Autodesk Inventor part; units mm, degrees
(part 2 of 2)
  spline S317 degree 2 poles (4.7592, -20.8202) (4.7075, -20.8826) (4.5777, -20.9876) knots 0 0 0 1 1 1
  line L179 (4.5777, -20.9876) -> (6.0592, -20.5763)
  spline S318 degree 2 poles (6.0592, -20.5763) (6.2625, -20.5199) (6.4389, -20.3989) (6.5028, -20.1862) (6.4937, -19.9698) knots 0 0 0 1 2 3 3 3
  line L180 (6.4937, -19.9698) -> (6.4825, -19.778)
  line L181 (6.4825, -19.778) -> (6.6607, -19.7285)
  spline S319 degree 2 poles (8.7637, -20.3753) (8.3867, -20.5516) (7.5473, -20.4146) (6.8295, -19.8283) (6.6188, -19.378) knots 0 0 0 1 2 3 3 3
  spline S320 degree 2 poles (6.6188, -19.378) (6.4106, -18.933) (6.4141, -18.006) (6.8248, -17.281) (7.2018, -17.1047) knots 0 0 0 1 2 3 3 3
  spline S321 degree 2 poles (7.2018, -17.1047) (7.3484, -17.0361) (7.7003, -16.9768) (8.0756, -17.015) (8.2787, -17.1082) knots 0 0 0 1 2 3 3 3
  spline S322 degree 2 poles (8.2787, -17.1082) (8.5842, -17.1951) (9.1378, -17.7306) (9.3178, -18.1154) knots 0 0 0 1 2 2 2
  spline S323 degree 2 poles (9.3178, -18.1154) (9.4281, -18.351) (9.5371, -18.8297) (9.5213, -19.287) (9.3843, -19.7308) (9.2645, -19.9112) knots 0 0 0 1 2 3 4 4 4
  spline S324 degree 2 poles (9.2645, -19.9112) (9.0516, -20.2406) (8.7637, -20.3753) knots 0 0 0 1 1 1
  line L182 (7.3086, -18.7108) -> (7.5755, -19.2815)
  spline S325 degree 2 poles (7.5755, -19.2815) (7.867, -19.9045) (8.3959, -20.3463) (8.6603, -20.2226) knots 0 0 0 1 2 2 2
  spline S326 degree 2 poles (8.6603, -20.2226) (9.1865, -19.9764) (8.6759, -18.8848) knots 0 0 0 1 1 1
  line L183 (8.6759, -18.8848) -> (8.4003, -18.2958)
  spline S327 degree 2 poles (8.4003, -18.2958) (8.2827, -18.0444) (8.0517, -17.6324) (7.9802, -17.5478) knots 0 0 0 1 2 2 2
  spline S328 degree 2 poles (7.9802, -17.5478) (7.6465, -17.1072) (7.28, -17.2787) knots 0 0 0 1 1 1
  spline S329 degree 2 poles (7.28, -17.2787) (7.0967, -17.3644) (6.978, -17.704) (7.1028, -18.271) (7.3086, -18.7108) knots 0 0 0 1 2 3 3 3
  line L184 (11.9387, -16.7133) -> (12.5299, -18.012)
  line L185 (12.5299, -18.012) -> (10.3324, -19.5294)
  spline S330 degree 2 poles (10.3324, -19.5294) (10.1686, -19.2668) (10.2153, -18.8411) knots 0 0 0 1 1 1
  spline S331 degree 2 poles (10.2153, -18.8411) (10.2457, -18.5392) (10.5063, -17.8078) knots 0 0 0 1 1 1
  spline S332 degree 2 poles (10.5063, -17.8078) (10.6457, -17.4094) (10.6659, -17.3217) knots 0 0 0 1 1 1
  spline S333 degree 2 poles (10.6659, -17.3217) (10.6697, -17.312) (10.6809, -17.2621) (10.6898, -17.2139) knots 0 0 0 1 2 2 2
  spline S334 degree 2 poles (10.6898, -17.2139) (10.7351, -16.9438) (10.6498, -16.5355) (10.5135, -16.3381) knots 0 0 0 1 2 2 2
  spline S335 degree 2 poles (10.5135, -16.3381) (10.282, -16.0028) (9.7155, -15.8742) (9.4182, -16.0795) knots 0 0 0 1 2 2 2
  spline S336 degree 2 poles (9.4182, -16.0795) (9.1875, -16.2388) (8.932, -16.6927) (8.9316, -17.1601) (9.0613, -17.348) knots 0 0 0 1 2 3 3 3
  spline S337 degree 2 poles (9.0613, -17.348) (9.1845, -17.5263) (9.2392, -17.4886) knots 0 0 0 1 1 1
  spline S338 degree 2 poles (9.2392, -17.4886) (9.2416, -17.4869) (9.2242, -17.4567) knots 0 0 0 1 1 1
  spline S339 degree 2 poles (9.2242, -17.4567) (9.1985, -17.4042) (9.1838, -17.3371) knots 0 0 0 1 1 1
  spline S340 degree 2 poles (9.1838, -17.3371) (9.148, -17.1581) (9.2472, -16.9) (9.3851, -16.8047) knots 0 0 0 1 2 2 2
  spline S341 degree 2 poles (9.3851, -16.8047) (9.4993, -16.7259) (9.7514, -16.6993) (9.9737, -16.8127) (10.0476, -16.9198) knots 0 0 0 1 2 3 3 3
  spline S342 degree 2 poles (10.0476, -16.9198) (10.1347, -17.0458) (10.1482, -17.335) (10.013, -17.597) (9.8798, -17.6889) knots 0 0 0 1 2 3 3 3
  spline S343 degree 2 poles (9.8798, -17.6889) (9.6349, -17.8581) (9.0877, -17.7372) (8.9087, -17.4779) knots 0 0 0 1 2 2 2
  spline S344 degree 2 poles (8.9087, -17.4779) (8.802, -17.3233) (8.7156, -16.9439) (8.7696, -16.717) knots 0 0 0 1 2 2 2
  spline S345 degree 2 poles (8.7696, -16.717) (8.8426, -16.2276) (9.468, -15.7956) knots 0 0 0 1 1 1
  spline S346 degree 2 poles (9.468, -15.7956) (9.7249, -15.6183) (10.2567, -15.4372) (10.7436, -15.4557) (11.1422, -15.6616) (11.2719, -15.8495) knots 0 0 0 1 2 3 4 4 4
  spline S347 degree 2 poles (11.2719, -15.8495) (11.4657, -16.1301) (11.422, -16.494) knots 0 0 0 1 1 1
  spline S348 degree 2 poles (11.422, -16.494) (11.4098, -16.6289) (11.3538, -16.787) knots 0 0 0 1 1 1
  spline S349 degree 2 poles (11.3538, -16.787) (11.2506, -17.0444) (10.973, -17.4714) knots 0 0 0 1 1 1
  spline S350 degree 2 poles (10.973, -17.4714) (10.5939, -18.0669) (10.4994, -18.3675) knots 0 0 0 1 1 1
  spline S351 degree 2 poles (10.4994, -18.3675) (10.471, -18.4433) (10.3827, -18.585) knots 0 0 0 1 1 1
  line L186 (10.3827, -18.585) -> (11.6479, -17.7113)
  spline S352 degree 2 poles (11.6479, -17.7113) (11.8215, -17.5914) (11.9486, -17.4194) (11.9394, -17.1975) (11.8599, -16.9959) knots 0 0 0 1 2 3 3 3
  line L187 (11.8599, -16.9959) -> (11.7864, -16.8184)
  line L188 (11.7864, -16.8184) -> (11.9387, -16.7133)
  spline S353 degree 2 poles (14.1375, -16.6358) (13.839, -16.9259) (13.001, -17.0713) (12.1308, -16.7523) (11.7843, -16.3959) knots 0 0 0 1 2 3 3 3
  spline S354 degree 2 poles (11.7843, -16.3959) (11.4419, -16.0435) (11.1417, -15.1665) (11.2923, -14.347) (11.5908, -14.057) knots 0 0 0 1 2 3 3 3
  spline S355 degree 2 poles (11.5908, -14.057) (11.7068, -13.9442) (12.0199, -13.7728) (12.387, -13.6861) (12.6095, -13.7077) knots 0 0 0 1 2 3 3 3
  spline S356 degree 2 poles (12.6095, -13.7077) (12.9266, -13.6897) (13.625, -14.0144) (13.9211, -14.3191) knots 0 0 0 1 2 2 2
  spline S357 degree 2 poles (13.9211, -14.3191) (14.1024, -14.5056) (14.3622, -14.9222) (14.497, -15.3594) (14.5129, -15.8236) (14.4588, -16.0334) knots 0 0 0 1 2 3 4 4 4
  spline S358 degree 2 poles (14.4588, -16.0334) (14.3655, -16.4142) (14.1375, -16.6358) knots 0 0 0 1 1 1
  line L189 (12.2176, -15.5395) -> (12.6567, -15.9913)
  spline S359 degree 2 poles (12.6567, -15.9913) (13.1361, -16.4846) (13.7805, -16.7288) (13.9898, -16.5254) knots 0 0 0 1 2 2 2
  spline S360 degree 2 poles (13.9898, -16.5254) (14.4064, -16.1205) (13.5665, -15.2562) knots 0 0 0 1 1 1
  line L190 (13.5665, -15.2562) -> (13.1132, -14.7899)
  spline S361 degree 2 poles (13.1132, -14.7899) (12.9199, -14.5909) (12.5666, -14.2773) (12.4714, -14.2208) knots 0 0 0 1 2 2 2
  spline S362 degree 2 poles (12.4714, -14.2208) (12.0118, -13.9138) (11.7216, -14.1958) knots 0 0 0 1 1 1
  spline S363 degree 2 poles (11.7216, -14.1958) (11.5766, -14.3368) (11.5755, -14.6965) (11.8791, -15.1913) (12.2176, -15.5395) knots 0 0 0 1 2 3 3 3
  point P0 (0, 0)
  point P1 (-50, 12.5)
  point P2 (-50, -12.5)
  dimension "d18" = 47.5
  dimension "d19" = 95
  constraints: 6 end point, 4 point on circle, 2 centre point, 2 horizontal, 2 other
  measures "d18" distance of L2.start L2.end
  measures "d19" distance of L2.end L3.end
extrude "Extrusion3" add sketch "Skizze3" against normal blind 2 from surface at -3
extrude "Extrusion4" add sketch "Skizze4" along normal blind 2
ref_plane "Arbeitsebene1" through (0, 0, 3) normal (0, 0, 1) x (1, 0, 0)
sketch "Skizze5" plane through (0, 0, 3) normal (0, 0, 1) x (1, 0, 0)
  line L0 (-8.4237, 9.7925) -> (8.4237, 9.7925)
  line L1 (8.4237, 9.7925) -> (8.4237, 8.1078)
  line L2 (8.4237, 8.1078) -> (-8.4237, 8.1078)
  line L3 (-8.4237, 8.1078) -> (-8.4237, 9.7925)
  line L4 (-8.4237, 9.7925) -> (8.4237, 8.1078) construction
  line L5 (8.4237, 9.7925) -> (-8.4237, 8.1078) construction
  line L6 (-8.4237, -10.2137) -> (8.4237, -10.2137)
  line L7 (8.4237, -10.2137) -> (8.4237, -11.8985)
  line L8 (8.4237, -11.8985) -> (-8.4237, -11.8985)
  line L9 (-8.4237, -11.8985) -> (-8.4237, -10.2137)
  line L10 (-8.4237, -10.2137) -> (8.4237, -11.8985) construction
  line L11 (8.4237, -10.2137) -> (-8.4237, -11.8985) construction
  point P0 (0, 0)
  point P1 (0, 8.9502)
  point P2 (0, -11.0561)
  constraints: 24 end point, 4 midpoint, 4 parallel, 2 horizontal, 2 perpendicular, 1 point on line
extrude "Extrusion5" add sketch "Skizze5" along normal blind 2
